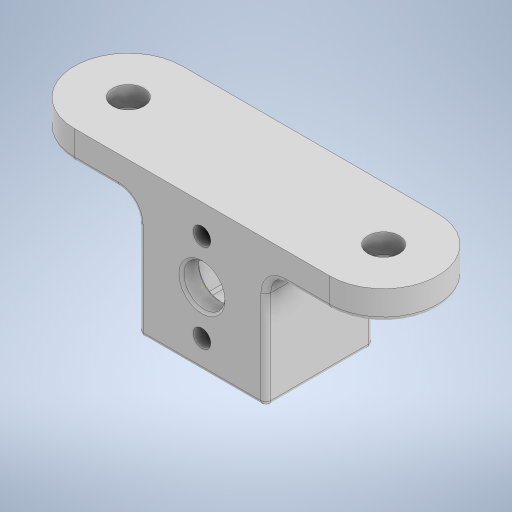
# Autodesk Inventor part: v2motormount
Saved by Autodesk Inventor 2024.2 (Build 282272000, 272)
## iProperties
Created: 2023-12-09
Part Number: v2motormount
Material: Generic
Document SubType Name: Modeling
Designer: Eric
Density: 1 g/cm^3
Appearance: Default
Author: Eric
Autodesk Inventor part; units mm, degrees
ref_plane "YZ Plane" through (0, 0, 0) normal (1, 0, 0) x (0, 1, 0)
ref_plane "XZ Plane" through (0, 0, 0) normal (0, 1, 0) x (-1, 0, 0)
ref_plane "XY Plane" through (0, 0, 0) normal (0, 0, 1) x (1, 0, 0)
sketch "Sketch1" plane through (0, 0, 0) normal (0, 1, 0) x (-1, 0, 0)
  point P0 (0, 0)
sketch "Sketch2" plane through (0, 0, 0) normal (0, 0, 1) x (1, 0, 0)
  circle A0 centre (0, -4.5) radius 0.9
  circle A1 centre (0, 4.5) radius 0.9
  circle A2 centre (0, 0) radius 2.0975
  line L0 (6.5, 7.5) -> (-6.5, 7.5)
  line L1 (-6.5, 7.5) -> (-6.5, -7.5)
  line L2 (-6.5, -7.5) -> (6.5, -7.5)
  line L3 (6.5, -7.5) -> (6.5, 7.5)
  dimension "d0" = 1.8
  dimension "d1" = 9
  dimension "d2" = 4.195
  dimension "d3" = 4.5
  dimension "d4" = 13
  dimension "d5" = 15
  dimension "d6" = 7.5
  dimension "d7" = 6.5
  constraints: 8 end point, 3 centre point, 2 parallel, 2 vertical alignment, 1 coincident, 1 equal radius, 1 horizontal, 1 perpendicular
  measures "d0" diameter of A1
  measures "d1" distance of A1.centre A0.centre
  measures "d2" diameter of A2
  measures "d3" distance of point (0, 0) A1.centre
  measures "d4" distance of L1.end L2.end
  measures "d5" distance of L2.end L0.start
  measures "d6" distance from line of point (0, 0) L0
  measures "d7" distance from line of point (0, 0) L3
extrude "Extrusion1" add sketch "Sketch2" against normal blind 2
sketch "Sketch3" plane through (0, 0, -2) normal (0, 0, -1) x (-1, 0, 0)
  line L0 (6.5, 7.5) -> (-6.5, 7.5) projected
  line L1 (-6.5, 7.5) -> (-6.5, -7.5) projected
  line L2 (6.5, -7.5) -> (6.5, 7.5) projected
  line L3 (-6.5, -7.5) -> (6.5, -7.5) projected
  line L4 (-5, 6) -> (5, 6)
  line L5 (5, 6) -> (5, -6)
  line L6 (5, -6) -> (-5, -6)
  line L7 (-5, -6) -> (-5, 6)
  point P0 (0, 0)
  dimension "d10" = 1.5
  dimension "d11" = 1.5
  dimension "d12" = 1.5
  dimension "d13" = 1.5
  constraints: 8 end point, 2 parallel, 1 horizontal, 1 perpendicular
  measures "d10" distance between parallel lines of L3 L6
  measures "d11" distance between parallel lines of L2 L5
  measures "d12" distance between parallel lines of L1 L7
  measures "d13" distance between parallel lines of L4 L0
extrude "Extrusion2" add sketch "Sketch3" along normal blind 9
sketch "Sketch4" plane through (-6.5, 7.5, 0) normal (0, 1, 0) x (1, 0, 0)
  line L0 (13, 11) -> (0, 11) projected
  line L1 (0, 11) -> (-12, 11)
  line L2 (-12, 11) -> (-12, 0)
  line L3 (0, 0) -> (13, 0) projected
  line L4 (-12, 0) -> (0, 0)
  line L5 (13, 0) -> (25, 0)
  line L6 (25, 0) -> (25, 11)
  line L7 (25, 11) -> (13, 11)
  line L8 (0, 0) -> (0, 11) projected
  line L9 (13, 0) -> (13, 11) projected
  circle A0 centre (-6.5, 5.5) radius 1.6
  circle A1 centre (19.5, 5.5) radius 1.6
  point P0 (6.5, 0)
  point P1 (-12, 5.5)
  point P2 (-6, 0)
  point P3 (19, 0)
  dimension "d16" = 3.2
  dimension "d17" = 12
  dimension "d22" = 5.5
  dimension "d23" = 5.5
  constraints: 12 end point, 3 midpoint, 3 perpendicular, 2 centre point, 2 collinear, 2 horizontal, 2 horizontal alignment, 1 equal radius
  measures "d16" diameter of A0
  measures "d17" distance between parallel lines of L8 L2
  measures "d22" distance from line of L2 A0.centre
  measures "d23" distance from line of L6 A1.centre
extrude "Extrusion3" add sketch "Sketch4" against normal blind 3 contours L7 L6 L5 L9 | L8 L4 L2 L1
fillet "Fillet1" radius 2 2 edges at (-6.5, 4.5, -5.5) (6.5, 4.5, -5.5)
fillet "Fillet2" radius 5.5 4 edges at (-18.5, 6, 0) (-18.5, 6, -11) (18.5, 6, 0) (18.5, 6, -11)
sketch "Sketch5" plane through (-6.5, 4.5, 0) normal (0, -1, 0) x (1, 0, 0)
  circle A0 centre (19.5, -5.5) radius 1.6 projected
  circle A1 centre (-6.5, -5.5) radius 1.6 projected
  circle A2 centre (19.5, -5.5) radius 2.55
  circle A3 centre (-6.5, -5.5) radius 2.55
  point P0 (6.5, 0)
  dimension "d24" = 5.1
  constraints: 2 centre point, 2 coincident, 1 equal radius
  measures "d24" diameter of A2
extrude "Extrusion4" cut sketch "Sketch5" against normal blind 1
fillet "Fillet3" radius 0.5 22 edges at (-6.5, -7.5, -5.5) (6.5, -7.5, -5.5) (-7.0858, 3.9142, 0) (-10.7501, 4.5, 0) (-16.8891, 4.5, -9.3891) (-16.8891, 4.5, -1.6109) (-18.5, 4.5, -5.5) (-10.7501, 4.5, -11) (-7.0858, 3.9142, -11) (-6.5, -2.5, -11) (-6.5, -2.5, 0) (7.0858, 3.9142, 0) (10.7501, 4.5, 0) (16.8891, 4.5, -1.6109) (18.5, 4.5, -5.5) (16.8891, 4.5, -9.3891) (10.7501, 4.5, -11) (7.0858, 3.9142, -11) (6.5, -2.5, -11) (6.5, -2.5, 0) (0, -7.5, 0) (0, -7.5, -11)
fillet "Fillet4" radius 0.25 4 edges at (5, -6, -6.5) (-5, -6, -6.5) (5, 6, -6.5) (-5, 6, -6.5)
chamfer "Chamfer1" distance 0.25 angle 45 10 edges at (-2.0975, 0, -2) (-2.0975, 0, 0) (0, -6, -11) (4.9268, -5.9268, -11) (5, 0, -11) (4.9268, 5.9268, -11) (0, 6, -11) (-4.9268, 5.9268, -11) (-5, 0, -11) (-4.9268, -5.9268, -11)
body "Solid1"
